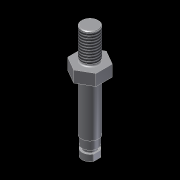
# Autodesk Inventor part: 移動輪固定軸
Saved by Autodesk Inventor 2012 SP1 (Build 160190100, 190)
## iProperties
Created: 2011-10-13
Part Number: 移動輪固定軸
Material: Default
Document SubType Name: Modeling
Designer: Eric
Density: 1 g/cm^3
Author: Eric
Autodesk Inventor part; units mm, degrees
sketch "草圖1" plane through (0, 0, 0) normal (0, 0, 1) x (1, 0, 0)
  line L0 (0, -11.547) -> (-10, -5.7735)
  line L1 (-10, -5.7735) -> (-10, 5.7735)
  line L2 (-10, 5.7735) -> (0, 11.547)
  line L3 (0, 11.547) -> (10, 5.7735)
  line L4 (10, 5.7735) -> (10, -5.7735)
  line L5 (10, -5.7735) -> (0, -11.547)
  point P0 (0, 0)
  point P1 (0, 0)
  dimension "d16" = 20
  constraints: 12 end point, 1 coincident, 13 other
  measures "d16" distance between parallel lines of L5 L2
extrude "擠出1" add sketch "草圖1" along normal blind 8
sketch "草圖2" plane through (0, 0, 8) normal (0, 0, 1) x (1, 0, 0)
  circle A0 centre (0, 0) radius 6
  dimension "d3" = 12
  constraints: 1 centre point, 1 coincident
  measures "d3" diameter of A0
extrude "擠出2" add sketch "草圖2" along normal blind 22
thread "螺紋1" size "M12x1.75" class "6g" standard "ANSI Metric M Profile" full length
sketch "草圖3" plane through (0, 0, 0) normal (0, 0, -1) x (-1, 0, 0)
  circle A0 centre (0, 0) radius 6
  dimension "d8" = 12
  constraints: 1 centre point, 1 coincident
  measures "d8" diameter of A0
extrude "擠出3" add sketch "草圖3" along normal blind 50
ref_plane "工作平面1" through (0, 0, -43) normal (0, 0, -1) x (-1, 0, 0)
sketch "草圖4" plane through (0, 0, -43) normal (0, 0, -1) x (-1, 0, 0)
  circle A0 centre (0, 0) radius 4.15
  circle A1 centre (0, 0) radius 6
  dimension "d12" = 8.3
  dimension "d13" = 12
  constraints: 2 centre point, 2 coincident
  measures "d12" diameter of A0
  measures "d13" diameter of A1
extrude "擠出4" cut sketch "草圖4" along normal blind 2.5
ref_plane "工作平面6" through (0, 0, 0) normal (0, 1, 0) x (-1, 0, 0)
chamfer "倒角1" distance 0.5 angle 45 1 edges at (-6, 0, 30)
ref_plane "工作平面8" through (0, 0, 0) normal (1, 0, 0) x (0, 1, 0)
sketch "草圖7" plane through (0, 0, 0) normal (1, 0, 0) x (0, 1, 0)
  line L0 (-5.5, 30) -> (5.5, 30) projected
  line L1 (-6, 8) -> (6, 8) projected
  line L2 (6, 29.5) -> (-6, 29.5) projected
  line L3 (-6, 8) -> (-6, 9)
  arc A0 (-6, 8) -> (-6, 10) centre (-6, 9) ccw
  line L4 (-6, 10) -> (-6, 8)
  line L5 (0, -6) -> (0, 36) projected
  point P0 (0, 0)
  constraints: 4 end point, 2 point on circle, 1 centre point, 1 coincident, 1 collinear, 1 perpendicular
revolve "迴轉1" cut sketch "草圖7" angle 360 about axis through (0, 0, -10) along (0, 0, 1)
sketch "草圖10" plane through (0, 0, -50) normal (0, 0, -1) x (-1, 0, 0)
  line L0 (-5, -2.2913) -> (-5, 2.2913)
  line L1 (5, 2.2913) -> (5, -2.2913)
  circle A0 centre (0, 0) radius 5.5 projected
  point P0 (5, -2.8868)
  point P1 (-5, -2.8868)
  point P2 (5, 2.8868)
  dimension "d40" = 10
  constraints: 4 end point, 4 point on circle, 3 point on line, 2 other
  measures "d40" distance between parallel lines of L0 L1
sketch "草圖11" plane through (0, 0, -50) normal (0, 0, -1) x (-1, 0, 0)
  arc A0 (6, 0) -> (6, 0) centre (0, 0) ccw projected
  circle A1 centre (0, 0) radius 5.5
  circle A2 centre (0, 0) radius 6
  dimension "d45" = 11
  constraints: 2 centre point, 2 coincident, 1 concentric
  measures "d45" diameter of A1
extrude "擠出10" cut sketch "草圖11" against normal blind 13
extrude "擠出11" cut sketch "草圖10" against normal up to next contours A0 L0 | L1 A0
